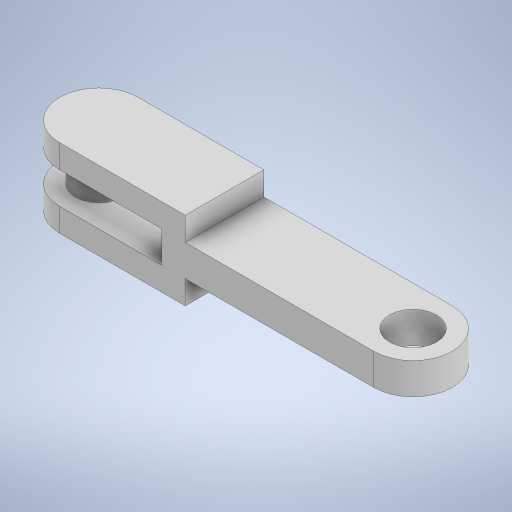
# Autodesk Inventor part: Manipulator Link
Saved by Autodesk Inventor 2023.2 (Build 272271030, 271C)
## iProperties
Created: 2023-06-26
Part Number: Manipulator Link
Material: Generic
Document SubType Name: Modeling
Designer: fist5
Density: 1 g/cm^3
Appearance: Default
Author: fist5
Autodesk Inventor part; units mm, degrees
ref_plane "YZ Plane" through (0, 0, 0) normal (1, 0, 0) x (0, 1, 0)
ref_plane "XZ Plane" through (0, 0, 0) normal (0, 1, 0) x (-1, 0, 0)
ref_plane "XY Plane" through (0, 0, 0) normal (0, 0, 1) x (1, 0, 0)
sketch "Sketch1" plane through (0, 0, 0) normal (0, 1, 0) x (-1, 0, 0)
  circle A0 centre (0, 0) radius 25
  circle A1 centre (-200, 0) radius 25
  line L0 (0, 25) -> (-200, 25)
  line L1 (-200, 25) -> (-200, -25)
  line L2 (-200, -25) -> (0, -25)
  line L3 (0, -25) -> (0, 25)
  point P0 (-200, 0)
  point P1 (0, 0)
  point P2 (0, -25)
  dimension "d0" = 50
  dimension "d1" = 50
  dimension "d2" = 200
  constraints: 8 end point, 3 horizontal, 2 midpoint, 2 parallel, 1 coincident, 1 horizontal alignment, 1 perpendicular, 6 other
  measures "d2" distance of point (-200, 0) point (0, 0)
extrude "Extrusion1" add sketch "Sketch1" along normal mid plane 20
sketch "Sketch4" plane through (0, 0, 0) normal (0, 1, 0) x (-1, 0, 0)
  arc A0 (0, -25) -> (0, 25) centre (0, 0) ccw projected
  line L0 (0, -25) -> (-200, -25) projected
  arc A1 (-200, 25) -> (-200, -25) centre (-200, 0) ccw projected
  line L1 (-200, 25) -> (0, 25) projected
  line L2 (0, -25) -> (-200, -25) projected
  line L3 (-80, -25) -> (-80, 25)
  line L4 (-200, 25) -> (0, 25) projected
  dimension "d10" = 80
  constraints: 2 end point, 2 point on line, 1 perpendicular
  measures "d10" distance from line of L3 point (0, 0)
extrude "Extrusion3" add sketch "Sketch4" along normal mid plane 50 contours L0 L3 L1 A0
sketch "Sketch6" plane through (0, 0, 0) normal (0, 1, 0) x (-1, 0, 0)
  circle A0 centre (0, 0) radius 15
  arc A1 (-200, 25) -> (-200, -25) centre (-200, 0) ccw projected
  circle A2 centre (-200, 0) radius 15
  line L0 (0, -25) -> (-80, -25) projected
  line L1 (-65, -25) -> (-65, 25)
  arc A3 (0, -25) -> (0, 25) centre (0, 0) ccw projected
  line L2 (-80, 25) -> (0, 25) projected
  point P0 (-65, 0)
  point P1 (25, 0)
  dimension "d13" = 30
  dimension "d14" = 30
  dimension "d16" = 90
  constraints: 2 centre point, 2 coincident, 2 end point, 1 horizontal alignment, 1 midpoint, 1 point on circle, 1 point on line, 1 vertical
  measures "d13" diameter of A0
  measures "d14" diameter of A2
  measures "d16" distance of point (-65, 0) point (25, 0)
extrude "Extrusion4" cut sketch "Sketch6" along normal mid plane 20
body "Solid1"
